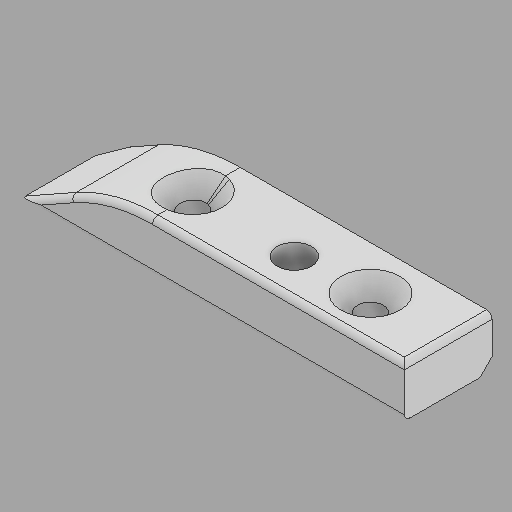
# Autodesk Inventor part: derz_LED
Saved by Autodesk Inventor 2024.2 (Build 282272000, 272)
## iProperties
Created: 2024-02-07
Part Number: derz_LED
Material: Типовые
Document SubType Name: Modeling
Designer: Fedor Orlov
Density: 1 g/cm^3
Appearance: По умолчанию
Author: Fedor Orlov
Autodesk Inventor part; units mm, degrees
ref_plane "YZ Plane" through (0, 0, 0) normal (1, 0, 0) x (0, 1, 0)
ref_plane "XZ Plane" through (0, 0, 0) normal (0, 1, 0) x (-1, 0, 0)
ref_plane "XY Plane" through (0, 0, 0) normal (0, 0, 1) x (1, 0, 0)
sketch "Эскиз1" plane through (0, 0, 0) normal (0, 1, 0) x (-1, 0, 0)
  line L0 (-13.3, -3.9495) -> (13.3, -3.9495)
  line L1 (13.3, -3.9495) -> (13.3, 3.9495)
  line L2 (13.3, 3.9495) -> (-13.3, 3.9495)
  line L3 (-13.3, 3.9495) -> (-13.3, -3.9495)
  line L4 (-13.3, -3.9495) -> (13.3, 3.9495) construction
  line L5 (13.3, -3.9495) -> (-13.3, 3.9495) construction
  line L6 (0, 3.9495) -> (0, -3.9495) construction
  circle A0 centre (0, 0.5505) radius 1.55
  circle A1 centre (-6.3, 0) radius 1.15
  circle A2 centre (9.7, 0) radius 1.15
  point P0 (0, 0)
  dimension "d0" = 13.3
  dimension "d1" = 7.899
  dimension "d2" = 3.1
  dimension "d3" = 4.5
  dimension "d35" = 2.3
  dimension "d36" = 2.3
  dimension "d37" = 7
  dimension "d38" = 16
  dimension "d39" = 3.9495
  dimension "d40" = 3.9495
  constraints: 14 end point, 4 midpoint, 3 centre point, 2 parallel, 1 horizontal, 1 perpendicular, 1 point on line
  measures "d0" distance from line of point (0, 0) L1
  measures "d1" distance of L0.end L1.end
  measures "d2" diameter of A0
  measures "d3" distance from line of A0.centre L0
  measures "d35" diameter of A1
  measures "d36" diameter of A2
  measures "d37" distance from line of L3 A1.centre
  measures "d38" distance of A1.centre A2.centre
  measures "d39" distance from line of L0 A2.centre
  measures "d40" distance from line of L0 A1.centre
extrude "Выдавливание1" add sketch "Эскиз1" along normal blind 4.5
sketch "Эскиз4" plane through (-13.3, 0, 3.9495) normal (0, 0, 1) x (1, 0, 0)
  line L0 (0, 0) -> (0, 4.5) projected
  line L1 (0, 0) -> (-8, 0)
  line L2 (0, 4.5) -> (26.6, 4.5) projected
  line L3 (-8, 0) -> (0, 4.5)
  point P0 (13.3, 0)
  point P1 (25.6, 4.5)
  point P2 (3.9103, 4.5)
  dimension "d19" = 8
  constraints: 4 end point, 1 horizontal
  measures "d19" distance of L0.start L1.end
extrude "Выдавливание4" add sketch "Эскиз4" against normal blind 7.899
fillet "Сопряжение4" radius 15 1 edges at (-13.3, 4.5, 0)
chamfer "Фаска2" distance 0.5 angle 45 1 edges at (1.55, 0, 0.5505)
chamfer "Фаска3" distance 1.1 angle 45 1 edges at (-4, 0, -3.9495)
fillet "Сопряжение7" radius 0.5 5 edges at (-4, 0, 3.9495) (-19.0123, 1.2868, 3.9495) (-13.1718, 4.0104, 3.9495) (1.9646, 4.5, 3.9495) (13.3, 4.5, 0)
chamfer "Фаска4" distance 1.5 angle 45 4 edges at (-8.55, 4.5, 0) (-10.4551, 4.4608, -0.8673) (-10.4603, 4.4604, 0.8628) (7.45, 4.5, 0)
equation "\"d39\" = 0.5 * d1"
equation "\"d40\" = d39"
